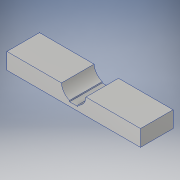
# Autodesk Inventor part: kfnmount
Saved by Autodesk Inventor 2019 (Build 230136000, 136)
## iProperties
Created: 2022-09-28
Part Number: kfnmount
Material: Aluminum 6061
Document SubType Name: Modeling
Designer: kananovicha
Density: 2.7 g/cm^3
Appearance: Aluminum - Flat
Author: kananovicha
Autodesk Inventor part; units mm, degrees
ref_plane "YZ Plane" through (0, 0, 0) normal (1, 0, 0) x (0, 1, 0)
ref_plane "XZ Plane" through (0, 0, 0) normal (0, 1, 0) x (-1, 0, 0)
ref_plane "XY Plane" through (0, 0, 0) normal (0, 0, 1) x (1, 0, 0)
sketch "Sketch1" plane through (0, 0, 0) normal (0, 0, 1) x (1, 0, 0)
  line L0 (-104.14, 12.7) -> (104.14, 12.7)
  line L1 (104.14, 12.7) -> (104.14, -12.7)
  line L2 (104.14, -12.7) -> (-104.14, -12.7)
  line L3 (-104.14, -12.7) -> (-104.14, 12.7)
  line L4 (-104.14, 12.7) -> (104.14, -12.7) construction
  line L5 (104.14, 12.7) -> (-104.14, -12.7) construction
  point P0 (0, 0)
  dimension "d0" = 208.28
  dimension "d1" = 25.4
  constraints: 12 end point, 2 midpoint, 2 parallel, 1 horizontal, 1 perpendicular
  measures "d0" distance of L1.end L2.end
  measures "d1" distance of L0.end L1.end
extrude "Extrusion1" add sketch "Sketch1" along normal mid plane 50.8
sketch "Sketch2" plane through (0, 0, 25.4) normal (0, 0, 1) x (1, 0, 0)
  line L0 (-104.14, 12.7) -> (-104.14, -12.7) projected
  line L1 (-104.14, -12.7) -> (104.14, -12.7) projected
  point P0 (0, 0)
  point P1 (0, 13.4938)
  dimension "d5" = 104.14
  dimension "d13" = 26.1938
  measures "d5" distance from line of point (0, 13.494) L0
  measures "d13" distance from line of point (0, 13.494) L1
hole "Hole1" at (0, 13.4938, 25.4) direction (0, 0, -1) diameter 38.1 end through all
sketch "Sketch3" plane through (0, 0, 25.4) normal (0, 0, 1) x (1, 0, 0)
  line L0 (-6.35, 12.7) -> (6.35, 12.7)
  line L1 (6.35, 12.7) -> (6.35, -6.35)
  line L2 (6.35, -6.35) -> (-6.35, -6.35)
  line L3 (-6.35, -6.35) -> (-6.35, 12.7)
  line L4 (104.14, 12.7) -> (19.0335, 12.7) projected
  line L5 (-104.14, 12.7) -> (-104.14, -12.7) projected
  point P0 (0, 0)
  dimension "d14" = 19.05
  dimension "d15" = 19.05
  dimension "d16" = 12.7
  dimension "d17" = 97.79
  constraints: 8 end point, 2 parallel, 1 horizontal, 1 perpendicular
  measures "d14" distance between parallel lines of L4 L2
  measures "d15" distance between parallel lines of L0 L2
  measures "d16" distance between parallel lines of L1 L3
  measures "d17" distance between parallel lines of L3 L5
extrude "Extrusion2" cut sketch "Sketch3" against normal through all
equation "\"d0\" = kn_wid"
equation "\"d1\" = kn_hei"
equation "\"d2\" = kn_len"
equation "\"d5\" = 0.5 * kn_wid"
equation "\"d13\" = kn_hei + kn_hole_offset"
equation "\"d6\" = kn_hole_diam"
equation "\"d14\" = kn_groove_hei"
equation "\"d15\" = kn_groove_hei"
equation "\"d16\" = kn_groove_wid"
equation "\"d17\" = 0.5 * kn_wid - 0.5 * kn_groove_wid"
equation "\"kn_wid\" = 208.28"
equation "\"kn_hei\" = 25.4"
equation "\"kn_len\" = 50.8"
equation "\"kn_hole_diam\" = 38.1"
equation "\"kn_groove_hei\" = 19.05"
equation "\"kn_groove_wid\" = 12.7"
equation "\"kn_hole_offset\" = 0.79375"
body "Solid1"
